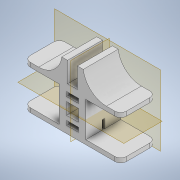
# Autodesk Inventor part: wing_honeycomb_interface
Saved by Autodesk Inventor 2021 (Build 250183000, 183)
## iProperties
Created: 2020-12-06
Part Number: wing_honeycomb_interface
Material: Generic
Document SubType Name: Modeling
Designer: victo
Density: 1 g/cm^3
Appearance: Default
Mass: 2.77932 g
Surface Area: 29.3964 cm^2
Volume: 2.77932 cm^3
Author: victo
Autodesk Inventor part; units mm, degrees
sketch "Sketch1" plane through (0, 0, 0) normal (0, 0, 1) x (1, 0, 0)
  line L0 (-4.55, 7.5) -> (4.55, 7.5)
  line L1 (4.55, 7.5) -> (4.55, -7.5)
  line L2 (4.55, -7.5) -> (-4.55, -7.5)
  line L3 (-4.55, -7.5) -> (-4.55, 7.5)
  line L4 (-4.55, 7.5) -> (4.55, -7.5) construction
  line L5 (4.55, 7.5) -> (-4.55, -7.5) construction
  line L6 (-2.05, -2.05) -> (2.05, -2.05)
  line L7 (2.05, -2.05) -> (2.05, 2.05)
  line L8 (2.05, 2.05) -> (-2.05, 2.05)
  line L9 (-2.05, 2.05) -> (-2.05, -2.05)
  line L10 (-2.05, -2.05) -> (2.05, 2.05) construction
  line L11 (2.05, -2.05) -> (-2.05, 2.05) construction
  line L12 (-4.55, 7.5) -> (-16.55, 7.5)
  line L13 (-16.55, 7.5) -> (-16.55, 6)
  line L14 (-16.55, 6) -> (-4.55, 6)
  line L15 (-4.55, 6) -> (-4.55, 7.5)
  line L16 (-4.55, -7.5) -> (-16.55, -7.5)
  line L17 (-16.55, -7.5) -> (-16.55, -6)
  line L18 (-16.55, -6) -> (-4.55, -6)
  line L19 (-4.55, -6) -> (-4.55, -7.5)
  line L20 (4.55, 7.5) -> (16.55, 7.5)
  line L21 (16.55, 7.5) -> (16.55, 6)
  line L22 (16.55, 6) -> (4.55, 6)
  line L23 (4.55, 6) -> (4.55, 7.5)
  line L24 (4.55, -7.5) -> (16.55, -7.5)
  line L25 (16.55, -7.5) -> (16.55, -6)
  line L26 (16.55, -6) -> (4.55, -6)
  line L27 (4.55, -6) -> (4.55, -7.5)
  point P0 (0, 0)
  point P1 (-4.55, 6)
  point P2 (-4.55, -6)
  point P3 (4.55, 6)
  dimension "d0" = 15
  dimension "d1" = 9.1
  dimension "d2" = 4.1
  dimension "d3" = 4.1
  dimension "d4" = 12
  dimension "d5" = 1.5
  dimension "d8" = 1.5
  dimension "d9" = 12
  dimension "d10" = 12
  dimension "d11" = 1.5
  dimension "d12" = 12
  constraints: 56 end point, 12 parallel, 6 horizontal, 6 perpendicular, 4 midpoint, 1 point on line
  measures "d0" distance of L0.end L1.end
  measures "d1" distance of L0.start L0.end
  measures "d2" distance of L7.end L8.end
  measures "d3" distance of L6.end L7.end
  measures "d4" distance of L21.end L22.end
  measures "d5" distance of L20.end L21.end
  measures "d8" distance of L16.end L17.end
  measures "d9" distance of L0.start L12.end
  measures "d10" distance of L17.end L18.end
  measures "d11" distance of L24.end L25.end
  measures "d12" distance of L25.end L26.end
extrude "Extrusion1" add sketch "Sketch1" along normal blind 12
sketch "Sketch2" plane through (0, 0, 12) normal (0, 0, 1) x (1, 0, 0)
  line L0 (16.55, 7.5) -> (-16.55, 7.5) projected
  line L1 (-3.7, 7.5) -> (-1.7, 7.5)
  line L2 (-1.7, 7.5) -> (-1.7, 14.5)
  line L3 (-1.7, 14.5) -> (-3.7, 14.5)
  line L4 (-3.7, 14.5) -> (-3.7, 7.5)
  line L5 (1.7, 7.5) -> (3.7, 7.5)
  line L6 (3.7, 7.5) -> (3.7, 14.5)
  line L7 (3.7, 14.5) -> (1.7, 14.5)
  line L8 (1.7, 14.5) -> (1.7, 7.5)
  point P0 (0, 0)
  dimension "d15" = 2
  dimension "d16" = 2
  dimension "d17" = 7
  dimension "d18" = 7
  dimension "d19" = 1.7
  dimension "d20" = 1.7
  constraints: 16 end point, 4 parallel, 2 horizontal, 2 perpendicular, 2 point on line
  measures "d15" distance of L6.end L7.end
  measures "d16" distance of L2.end L3.end
  measures "d17" distance of L1.end L2.end
  measures "d18" distance of L5.end L6.end
  measures "d19" distance from line of point (0, 0) L8
  measures "d20" distance from line of point (0, 0) L2
extrude "Extrusion2" add sketch "Sketch2" against normal up to surface (12 mm away)
fillet "Fillet1" radius 8 2 edges at (3.7, 7.5, 6) (-3.7, 7.5, 6)
sketch "Sketch3" plane through (4.55, -6, 0) normal (1, 0, 0) x (0, 0, -1)
  line L0 (-6.4, 3.1) -> (-5.6, 3.1)
  line L1 (-5.6, 3.1) -> (-5.6, 0)
  line L2 (-5.6, 0) -> (-6.4, 0)
  line L3 (-6.4, 0) -> (-6.4, 3.1)
  line L4 (0, 12) -> (-12, 12) projected
  line L5 (0, 0) -> (0, 12) projected
  line L6 (0, 0) -> (-12, 0) projected
  point P0 (0, 6)
  dimension "d24" = 3.1
  dimension "d25" = 0.8
  dimension "d30" = 0
  dimension "d39" = 12
  dimension "d40" = 5.6
  constraints: 8 end point, 2 parallel, 1 horizontal, 1 perpendicular
  measures "d24" distance of L0.end L1.end
  measures "d25" distance of L0.start L0.end
  measures "d30" distance between parallel lines of L6 L2
  measures "d39" distance of L5.start L6.end
  measures "d40" distance between parallel lines of L5 L1
extrude "Extrusion3" cut sketch "Sketch3" against normal through all
sketch "Sketch5" plane through (0, 0, 0) normal (0, 0, -1) x (-1, 0, 0)
  line L0 (-2.05, 5.05) -> (2.05, 5.05)
  line L1 (2.05, 5.05) -> (2.05, 3.55)
  line L2 (2.05, 3.55) -> (-2.05, 3.55)
  line L3 (-2.05, 3.55) -> (-2.05, 5.05)
  line L4 (-2.05, -3.55) -> (2.05, -3.55)
  line L5 (2.05, -3.55) -> (2.05, -5.05)
  line L6 (2.05, -5.05) -> (-2.05, -5.05)
  line L7 (-2.05, -5.05) -> (-2.05, -3.55)
  line L8 (2.05, 2.05) -> (-2.05, 2.05) projected
  line L9 (2.05, -2.05) -> (2.05, 2.05) projected
  line L10 (-2.05, -2.05) -> (2.05, -2.05) projected
  point P0 (0, 0)
  dimension "d31" = 4.1
  dimension "d32" = 4.1
  dimension "d33" = 1.5
  dimension "d34" = 1.5
  dimension "d35" = 1.5
  dimension "d36" = 1.5
  constraints: 16 end point, 4 parallel, 2 horizontal, 2 perpendicular, 2 point on line, 1 collinear
  measures "d31" distance of L0.start L0.end
  measures "d32" distance of L8.start L8.end
  measures "d33" distance between parallel lines of L8 L2
  measures "d34" distance of L0.end L1.end
  measures "d35" distance between parallel lines of L4 L10
  measures "d36" distance of L4.end L5.end
extrude "Extrusion4" cut sketch "Sketch5" against normal through all
fillet "Fillet2" radius 2 8 edges at (-16.55, 6.75, 0) (-16.55, 6.75, 12) (-16.55, -6.75, 0) (-16.55, -6.75, 12) (16.55, 6.75, 12) (16.55, -6.75, 12) (16.55, 6.75, 0) (16.55, -6.75, 0)
equation "\"d40\" = -0.5 * d25 + 0.5 * d39"
equation "\"d31\" = d32"
body "Solid1"
